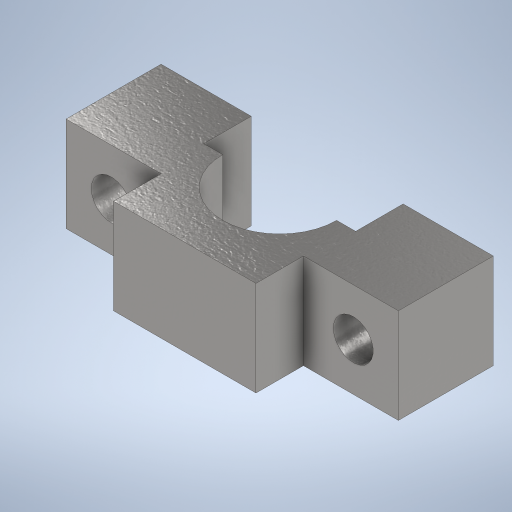
# Autodesk Inventor part: Pleuel_Unterteil
Saved by Autodesk Inventor 2024 (Build 280153000, 153)
## iProperties
Created: 2024-02-29
Part Number: Pleuel_Unterteil
Material: Stahl, galvanisiert
Document SubType Name: Modeling
Designer: ffogue
Density: 7.85 g/cm^3
Appearance: Galvanisiert
Author: ffogue
Autodesk Inventor part; units mm, degrees
ref_plane "YZ Plane" through (0, 0, 0) normal (1, 0, 0) x (0, 1, 0)
ref_plane "XZ Plane" through (0, 0, 0) normal (0, 1, 0) x (-1, 0, 0)
ref_plane "XY Plane" through (0, 0, 0) normal (0, 0, 1) x (1, 0, 0)
sketch "Skizze1" plane through (0, 0, 0) normal (0, 0, 1) x (1, 0, 0)
  line L0 (-17.5, 5) -> (-17.5, 15)
  line L1 (-17.5, 15) -> (-8, 15)
  line L2 (-8, 15) -> (-8, 10)
  line L3 (-8, 10) -> (8, 10)
  line L4 (8, 10) -> (8, 15)
  line L5 (8, 15) -> (17.5, 15)
  line L6 (17.5, 15) -> (17.5, 5)
  line L7 (-7.5, 5) -> (-17.5, 5)
  line L8 (0, 10) -> (0, 0) construction
  line L9 (17.5, 5) -> (7.5, 5)
  line L10 (7.5, 5) -> (7.5, 0)
  line L11 (-7.5, 0) -> (-7.5, 5)
  line L12 (-7.5, 0) -> (7.5, 0)
  point P0 (-12.75, 15)
  dimension "d0" = 16
  dimension "d1" = 5
  dimension "d2" = 35
  dimension "d7" = 15
  dimension "d10" = 5
  dimension "d11" = 15
  constraints: 26 end point, 7 perpendicular, 3 midpoint, 3 point on line, 1 coincident, 1 horizontal, 1 vertical, 2 other
  measures "d0" distance between parallel lines of L4 L2
  measures "d1" distance between parallel lines of L3 L1
  measures "d2" distance between parallel lines of L6 L0
  measures "d7" distance between parallel lines of L10 L11
  measures "d10" distance between parallel lines of L12 L7
  measures "d11" distance from line of L12 point (-12.75, 15)
extrude "Extrusion1" add sketch "Skizze1" along normal blind 10
sketch "Skizze2" plane through (0, 0, 10) normal (0, 0, 1) x (1, 0, 0)
  line L0 (8, 10) -> (-8, 10) projected
  arc A0 (-6, 10) -> (6, 10) centre (0, 10) ccw
  point P0 (0, 0)
  dimension "d12" = 6
  constraints: 2 point on circle, 2 point on line, 1 centre point, 1 coincident, 1 midpoint
  measures "d12" radius of A0
extrude "Extrusion2" cut sketch "Skizze2" against normal blind 10
sketch "Skizze3" plane through (-17.5, 15, 0) normal (0, 1, 0) x (1, 0, 0)
  line L0 (0, 0) -> (0, -10) projected
  line L1 (35, 0) -> (35, -10) projected
  line L2 (17.5, 0) -> (17.5, -10) construction
  point P0 (4.75, -5)
  point P1 (30.25, -5)
  point P2 (0, -5)
  point P3 (35, -5)
  dimension "d15" = 25.5
  constraints: 2 end point, 2 horizontal alignment, 2 midpoint, 1 symmetric about line, 1 vertical
  measures "d15" distance of point (30.25, -5) point (4.75, -5)
hole "Bohrung1" at (-12.75, 15, 5) at (12.75, 15, 5) direction (0, -1, 0) diameter 4.2 end through all
